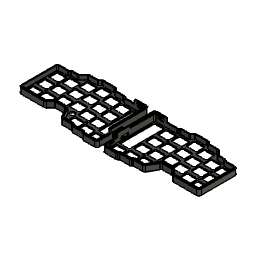
mriya-bumper-fdm-v1.09 (Autodesk Fusion 360 design; units mm, degrees)
Autodesk Fusion 360 part; units mm, degrees
note: some values were not read from the file. Set by a fixed rule: which sketch regions a step uses.
(part 1 of 2)
sketch "mriya" plane through (0, 0, 0) normal (0, 0, 1) x (1, 0, 0)
  line L0 (-101.0213, 15.6719) -> (-94.7787, 21.9145) construction
  line L1 (-26.4858, 1.079) -> (-27.6142, 2.2074) construction
  line L2 (-138.1, 14.7932) -> (-103.1426, 14.7932) construction
  line L3 (-44.0716, 2.7932) -> (-29.0284, 2.7932) construction
  line L4 (-8.6, 0.4932) -> (-25.0716, 0.4932) construction
  line L5 (-64.4741, 6.1094) -> (-72.7517, 20.7608) construction
  line L6 (-45.4858, 3.379) -> (-46.6142, 4.5074) construction
  line L7 (-122.6142, 71.579) -> (-121.4858, 72.7074) construction
  line L8 (-101.0716, 81.2932) -> (-87.2284, 81.2932) construction
  line L9 (-138.1, 70.9932) -> (-124.0284, 70.9932) construction
  line L10 (-92.6574, 22.7932) -> (-76.2344, 22.7932) construction
  line L11 (-48.0284, 5.0932) -> (-62.7328, 5.0932) construction
  line L12 (-82.0716, 84.7932) -> (-64.7284, 84.7932) construction
  line L13 (-58.5716, 80.2932) -> (-45.7284, 80.2932) construction
  line L14 (-24.1, 19.4932) -> (-7.1, 19.4932) construction
  line L15 (-25.6, 20.9932) -> (-25.6, 77.9932) construction
  line L16 (-83.4858, 84.2074) -> (-85.8142, 81.879) construction
  line L17 (-63.3142, 84.2074) -> (-59.9858, 80.879) construction
  line L18 (-139.6, 69.4932) -> (-139.6, 16.2932) construction
  line L19 (-43.1858, 78.579) -> (-44.3142, 79.7074) construction
  line L20 (-99.4, 40.3932) -> (-99.4, 27.9932) construction
  line L21 (-98.6, 41.1932) -> (-86.2, 41.1932) construction
  line L22 (-98.6, 27.1932) -> (-86.2, 27.1932) construction
  line L23 (-85.4, 40.3932) -> (-85.4, 27.9932) construction
  line L24 (-42.4, 56.0932) -> (-42.4, 43.6932) construction
  line L25 (-41.6, 56.8932) -> (-29.2, 56.8932) construction
  line L26 (-41.6, 42.8932) -> (-29.2, 42.8932) construction
  line L27 (-28.4, 56.0932) -> (-28.4, 43.6932) construction
  line L28 (-61.4, 58.3932) -> (-61.4, 45.9932) construction
  line L29 (-60.6, 59.1932) -> (-48.2, 59.1932) construction
  line L30 (-60.6, 45.1932) -> (-48.2, 45.1932) construction
  line L31 (-47.4, 58.3932) -> (-47.4, 45.9932) construction
  line L32 (-137.4, 68.0932) -> (-137.4, 55.6932) construction
  line L33 (-136.6, 68.8932) -> (-124.2, 68.8932) construction
  line L34 (-136.6, 54.8932) -> (-124.2, 54.8932) construction
  line L35 (-123.4, 68.0932) -> (-123.4, 55.6932) construction
  line L36 (-61.4, 39.3932) -> (-61.4, 26.9932) construction
  line L37 (-60.6, 40.1932) -> (-48.2, 40.1932) construction
  line L38 (-60.6, 26.1932) -> (-48.2, 26.1932) construction
  line L39 (-47.4, 39.3932) -> (-47.4, 26.9932) construction
  line L40 (-42.4, 18.0932) -> (-42.4, 5.6932) construction
  line L41 (-41.6, 18.8932) -> (-29.2, 18.8932) construction
  line L42 (-41.6, 4.8932) -> (-29.2, 4.8932) construction
  line L43 (-28.4, 18.0932) -> (-28.4, 5.6932) construction
  line L44 (-23.4, 15.7932) -> (-23.4, 3.3932) construction
  line L45 (-22.6, 16.5932) -> (-10.2, 16.5932) construction
  line L46 (-22.6, 2.5932) -> (-10.2, 2.5932) construction
  line L47 (-9.4, 15.7932) -> (-9.4, 3.3932) construction
  line L48 (-137.4, 49.0932) -> (-137.4, 36.6932) construction
  line L49 (-136.6, 49.8932) -> (-124.2, 49.8932) construction
  line L50 (-136.6, 35.8932) -> (-124.2, 35.8932) construction
  line L51 (-123.4, 49.0932) -> (-123.4, 36.6932) construction
  line L52 (-118.4, 51.3932) -> (-118.4, 38.9932) construction
  line L53 (-117.6, 52.1932) -> (-105.2, 52.1932) construction
  line L54 (-117.6, 38.1932) -> (-105.2, 38.1932) construction
  line L55 (-104.4, 51.3932) -> (-104.4, 38.9932) construction
  line L56 (-137.4, 30.0932) -> (-137.4, 17.6932) construction
  line L57 (-136.6, 30.8932) -> (-124.2, 30.8932) construction
  line L58 (-136.6, 16.8932) -> (-124.2, 16.8932) construction
  line L59 (-123.4, 30.0932) -> (-123.4, 17.6932) construction
  line L60 (-61.4, 20.3932) -> (-61.4, 7.9932) construction
  line L61 (-60.6, 21.1932) -> (-48.2, 21.1932) construction
  line L62 (-60.6, 7.1932) -> (-48.2, 7.1932) construction
  line L63 (-47.4, 20.3932) -> (-47.4, 7.9932) construction
  line L64 (-80.4, 43.8932) -> (-80.4, 31.4932) construction
  line L65 (-79.6, 44.6932) -> (-67.2, 44.6932) construction
  line L66 (-79.6, 30.6932) -> (-67.2, 30.6932) construction
  line L67 (-66.4, 43.8932) -> (-66.4, 31.4932) construction
  line L68 (-80.4, 81.8932) -> (-80.4, 69.4932) construction
  line L69 (-79.6, 82.6932) -> (-67.2, 82.6932) construction
  line L70 (-79.6, 68.6932) -> (-67.2, 68.6932) construction
  line L71 (-66.4, 81.8932) -> (-66.4, 69.4932) construction
  line L72 (-42.4, 37.0932) -> (-42.4, 24.6932) construction
  line L73 (-41.6, 37.8932) -> (-29.2, 37.8932) construction
  line L74 (-41.6, 23.8932) -> (-29.2, 23.8932) construction
  line L75 (-28.4, 37.0932) -> (-28.4, 24.6932) construction
  line L76 (-118.4, 32.3932) -> (-118.4, 19.9932) construction
  line L77 (-117.6, 33.1932) -> (-105.2, 33.1932) construction
  line L78 (-117.6, 19.1932) -> (-105.2, 19.1932) construction
  line L79 (-104.4, 32.3932) -> (-104.4, 19.9932) construction
  line L80 (-61.4, 77.3932) -> (-61.4, 64.9932) construction
  line L81 (-60.6, 78.1932) -> (-48.2, 78.1932) construction
  line L82 (-60.6, 64.1932) -> (-48.2, 64.1932) construction
  line L83 (-47.4, 77.3932) -> (-47.4, 64.9932) construction
  line L84 (-42.4, 75.0932) -> (-42.4, 62.6932) construction
  line L85 (-41.6, 75.8932) -> (-29.2, 75.8932) construction
  line L86 (-41.6, 61.8932) -> (-29.2, 61.8932) construction
  line L87 (-28.4, 75.0932) -> (-28.4, 62.6932) construction
  line L88 (-118.4, 70.3932) -> (-118.4, 57.9932) construction
  line L89 (-117.6, 71.1932) -> (-105.2, 71.1932) construction
  line L90 (-117.6, 57.1932) -> (-105.2, 57.1932) construction
  line L91 (-104.4, 70.3932) -> (-104.4, 57.9932) construction
  line L92 (-99.4, 59.3932) -> (-99.4, 46.9932) construction
  line L93 (-98.6, 60.1932) -> (-86.2, 60.1932) construction
  line L94 (-98.6, 46.1932) -> (-86.2, 46.1932) construction
  line L95 (-85.4, 59.3932) -> (-85.4, 46.9932) construction
  line L96 (-80.4, 62.8932) -> (-80.4, 50.4932) construction
  line L97 (-79.6, 63.6932) -> (-67.2, 63.6932) construction
  line L98 (-79.6, 49.6932) -> (-67.2, 49.6932) construction
  line L99 (-66.4, 62.8932) -> (-66.4, 50.4932) construction
  line L100 (-99.4, 78.3932) -> (-99.4, 65.9932) construction
  line L101 (-98.6, 79.1932) -> (-86.2, 79.1932) construction
  line L102 (-98.6, 65.1932) -> (-86.2, 65.1932) construction
  line L103 (-85.4, 78.3932) -> (-85.4, 65.9932) construction
  circle A0 centre (-120.9, 53.5432) radius 1.75
  circle A1 centre (-120.9, 34.5432) radius 1.75
  circle A2 centre (-68.5, 23.5932) radius 4
  circle A3 centre (-44.9, 22.5432) radius 1.75
  circle A4 centre (-44.9, 60.5432) radius 1.75
  arc A5 (-43.1858, 78.579) -> (-41.7716, 77.9932) centre (-41.7716, 79.9932) ccw construction
  arc A6 (-44.3142, 79.7074) -> (-45.7284, 80.2932) centre (-45.7285, 78.2931) ccw construction
  arc A7 (-59.9858, 80.879) -> (-58.5716, 80.2932) centre (-58.5716, 82.2931) ccw construction
  arc A8 (-63.3142, 84.2074) -> (-64.7284, 84.7932) centre (-64.7285, 82.7931) ccw construction
  arc A9 (-82.0716, 84.7932) -> (-83.4858, 84.2074) centre (-82.0716, 82.7933) ccw construction
  arc A10 (-87.2284, 81.2932) -> (-85.8142, 81.879) centre (-87.2284, 83.2932) ccw construction
  arc A11 (-101.0716, 81.2932) -> (-102.4858, 80.7074) centre (-101.0716, 79.2933) ccw construction
  arc A12 (-120.0716, 73.2932) -> (-121.4858, 72.7074) centre (-120.0716, 71.2933) ccw construction
  arc A13 (-124.0284, 70.9932) -> (-122.6142, 71.579) centre (-124.0284, 72.9932) ccw construction
  arc A14 (-138.1, 70.9932) -> (-139.6, 69.4932) centre (-138.1, 69.4932) ccw construction
  arc A15 (-139.6, 16.2932) -> (-138.1, 14.7932) centre (-138.1, 16.2932) ccw construction
  arc A16 (-103.1426, 14.7932) -> (-101.0213, 15.6719) centre (-103.1426, 17.7931) ccw construction
  arc A17 (-92.6574, 22.7932) -> (-94.7787, 21.9145) centre (-92.6573, 19.7931) ccw construction
  arc A18 (-72.7517, 20.7608) -> (-76.2344, 22.7932) centre (-76.2344, 18.793) ccw construction
  arc A19 (-64.4741, 6.1094) -> (-62.7328, 5.0932) centre (-62.7328, 7.0932) ccw construction
  arc A20 (-46.6142, 4.5074) -> (-48.0284, 5.0932) centre (-48.0284, 3.0933) ccw construction
  arc A21 (-45.4858, 3.379) -> (-44.0716, 2.7932) centre (-44.0715, 4.7933) ccw construction
  arc A22 (-27.6142, 2.2074) -> (-29.0284, 2.7932) centre (-29.0284, 0.7933) ccw construction
  arc A23 (-26.4858, 1.079) -> (-25.0716, 0.4932) centre (-25.0715, 2.4933) ccw construction
  arc A24 (-8.6, 0.4932) -> (-7.1, 1.9932) centre (-8.6, 1.9932) ccw construction
  arc A25 (-25.6, 20.9932) -> (-24.1, 19.4932) centre (-24.1, 20.9932) ccw construction
  line L104 (-7.1, 1.9932) -> (-7.1, 76.4932) construction
  line L105 (-41.7716, 77.9932) -> (-8.6, 77.9932) construction
  arc A26 (-7.1, 76.4932) -> (-8.6, 77.9932) centre (-8.6, 76.4932) ccw construction
  arc A27 (-136.6, 68.8932) -> (-137.4, 68.0932) centre (-136.6, 68.0932) ccw construction
  arc A28 (-123.4, 68.0932) -> (-124.2, 68.8932) centre (-124.2, 68.0932) ccw construction
  arc A29 (-124.2, 54.8932) -> (-123.4, 55.6932) centre (-124.2, 55.6932) ccw construction
  arc A30 (-137.4, 55.6932) -> (-136.6, 54.8932) centre (-136.6, 55.6932) ccw construction
  arc A31 (-136.6, 49.8932) -> (-137.4, 49.0932) centre (-136.6, 49.0932) ccw construction
  arc A32 (-123.4, 49.0932) -> (-124.2, 49.8932) centre (-124.2, 49.0932) ccw construction
  arc A33 (-124.2, 35.8932) -> (-123.4, 36.6932) centre (-124.2, 36.6932) ccw construction
  arc A34 (-137.4, 36.6932) -> (-136.6, 35.8932) centre (-136.6, 36.6932) ccw construction
  arc A35 (-136.6, 30.8932) -> (-137.4, 30.0932) centre (-136.6, 30.0932) ccw construction
  arc A36 (-123.4, 30.0932) -> (-124.2, 30.8932) centre (-124.2, 30.0932) ccw construction
  arc A37 (-124.2, 16.8932) -> (-123.4, 17.6932) centre (-124.2, 17.6932) ccw construction
  arc A38 (-137.4, 17.6932) -> (-136.6, 16.8932) centre (-136.6, 17.6932) ccw construction
  arc A39 (-118.4, 19.9932) -> (-117.6, 19.1932) centre (-117.6, 19.9932) ccw construction
  arc A40 (-105.2, 19.1932) -> (-104.4, 19.9932) centre (-105.2, 19.9932) ccw construction
  arc A41 (-104.4, 32.3932) -> (-105.2, 33.1932) centre (-105.2, 32.3932) ccw construction
  arc A42 (-117.6, 33.1932) -> (-118.4, 32.3932) centre (-117.6, 32.3932) ccw construction
  arc A43 (-105.2, 38.1932) -> (-104.4, 38.9932) centre (-105.2, 38.9932) ccw construction
  arc A44 (-118.4, 38.9932) -> (-117.6, 38.1932) centre (-117.6, 38.9932) ccw construction
  arc A45 (-117.6, 52.1932) -> (-118.4, 51.3932) centre (-117.6, 51.3932) ccw construction
  arc A46 (-104.4, 51.3932) -> (-105.2, 52.1932) centre (-105.2, 51.3932) ccw construction
  arc A47 (-118.4, 57.9932) -> (-117.6, 57.1932) centre (-117.6, 57.9932) ccw construction
  arc A48 (-105.2, 57.1932) -> (-104.4, 57.9932) centre (-105.2, 57.9932) ccw construction
  arc A49 (-104.4, 70.3932) -> (-105.2, 71.1932) centre (-105.2, 70.3932) ccw construction
  arc A50 (-117.6, 71.1932) -> (-118.4, 70.3932) centre (-117.6, 70.3932) ccw construction
  arc A51 (-98.6, 79.1932) -> (-99.4, 78.3932) centre (-98.6, 78.3932) ccw construction
  arc A52 (-85.4, 78.3932) -> (-86.2, 79.1932) centre (-86.2, 78.3932) ccw construction
  arc A53 (-86.2, 65.1932) -> (-85.4, 65.9932) centre (-86.2, 65.9932) ccw construction
  arc A54 (-99.4, 65.9932) -> (-98.6, 65.1932) centre (-98.6, 65.9932) ccw construction
  arc A55 (-98.6, 60.1932) -> (-99.4, 59.3932) centre (-98.6, 59.3932) ccw construction
  arc A56 (-85.4, 59.3932) -> (-86.2, 60.1932) centre (-86.2, 59.3932) ccw construction
  arc A57 (-86.2, 46.1932) -> (-85.4, 46.9932) centre (-86.2, 46.9932) ccw construction
  arc A58 (-99.4, 46.9932) -> (-98.6, 46.1932) centre (-98.6, 46.9932) ccw construction
  arc A59 (-98.6, 41.1932) -> (-99.4, 40.3932) centre (-98.6, 40.3932) ccw construction
  arc A60 (-99.4, 27.9932) -> (-98.6, 27.1932) centre (-98.6, 27.9932) ccw construction
  arc A61 (-86.2, 27.1932) -> (-85.4, 27.9932) centre (-86.2, 27.9932) ccw construction
  arc A62 (-85.4, 40.3932) -> (-86.2, 41.1932) centre (-86.2, 40.3932) ccw construction
  arc A63 (-80.4, 31.4932) -> (-79.6, 30.6932) centre (-79.6, 31.4932) ccw construction
  arc A64 (-79.6, 44.6932) -> (-80.4, 43.8932) centre (-79.6, 43.8932) ccw construction
  arc A65 (-66.4, 43.8932) -> (-67.2, 44.6932) centre (-67.2, 43.8932) ccw construction
  arc A66 (-67.2, 30.6932) -> (-66.4, 31.4932) centre (-67.2, 31.4932) ccw construction
  arc A67 (-67.2, 49.6932) -> (-66.4, 50.4932) centre (-67.2, 50.4932) ccw construction
  arc A68 (-80.4, 50.4932) -> (-79.6, 49.6932) centre (-79.6, 50.4932) ccw construction
  arc A69 (-79.6, 63.6932) -> (-80.4, 62.8932) centre (-79.6, 62.8932) ccw construction
  arc A70 (-66.4, 62.8932) -> (-67.2, 63.6932) centre (-67.2, 62.8932) ccw construction
  arc A71 (-67.2, 68.6932) -> (-66.4, 69.4932) centre (-67.2, 69.4932) ccw construction
  arc A72 (-80.4, 69.4932) -> (-79.6, 68.6932) centre (-79.6, 69.4932) ccw construction
  arc A73 (-79.6, 82.6932) -> (-80.4, 81.8932) centre (-79.6, 81.8932) ccw construction
  arc A74 (-66.4, 81.8932) -> (-67.2, 82.6932) centre (-67.2, 81.8932) ccw construction
  arc A75 (-60.6, 78.1932) -> (-61.4, 77.3932) centre (-60.6, 77.3932) ccw construction
  arc A76 (-61.4, 64.9932) -> (-60.6, 64.1932) centre (-60.6, 64.9932) ccw construction
  arc A77 (-48.2, 64.1932) -> (-47.4, 64.9932) centre (-48.2, 64.9932) ccw construction
  arc A78 (-47.4, 77.3932) -> (-48.2, 78.1932) centre (-48.2, 77.3932) ccw construction
  arc A79 (-47.4, 58.3932) -> (-48.2, 59.1932) centre (-48.2, 58.3932) ccw construction
  arc A80 (-60.6, 59.1932) -> (-61.4, 58.3932) centre (-60.6, 58.3932) ccw construction
  arc A81 (-61.4, 45.9932) -> (-60.6, 45.1932) centre (-60.6, 45.9932) ccw construction
  arc A82 (-48.2, 45.1932) -> (-47.4, 45.9932) centre (-48.2, 45.9932) ccw construction
  arc A83 (-47.4, 39.3932) -> (-48.2, 40.1932) centre (-48.2, 39.3932) ccw construction
  arc A84 (-60.6, 40.1932) -> (-61.4, 39.3932) centre (-60.6, 39.3932) ccw construction
  arc A85 (-61.4, 26.9932) -> (-60.6, 26.1932) centre (-60.6, 26.9932) ccw construction
  arc A86 (-48.2, 26.1932) -> (-47.4, 26.9932) centre (-48.2, 26.9932) ccw construction
  arc A87 (-47.4, 20.3932) -> (-48.2, 21.1932) centre (-48.2, 20.3932) ccw construction
  arc A88 (-60.6, 21.1932) -> (-61.4, 20.3932) centre (-60.6, 20.3932) ccw construction
  arc A89 (-61.4, 7.9932) -> (-60.6, 7.1932) centre (-60.6, 7.9932) ccw construction
  arc A90 (-48.2, 7.1932) -> (-47.4, 7.9932) centre (-48.2, 7.9932) ccw construction
  arc A91 (-42.4, 5.6932) -> (-41.6, 4.8932) centre (-41.6, 5.6932) ccw construction
  arc A92 (-29.2, 4.8932) -> (-28.4, 5.6932) centre (-29.2, 5.6932) ccw construction
  arc A93 (-28.4, 18.0932) -> (-29.2, 18.8932) centre (-29.2, 18.0932) ccw construction
  arc A94 (-41.6, 18.8932) -> (-42.4, 18.0932) centre (-41.6, 18.0932) ccw construction
  arc A95 (-23.4, 3.3932) -> (-22.6, 2.5932) centre (-22.6, 3.3932) ccw construction
  arc A96 (-10.2, 2.5932) -> (-9.4, 3.3932) centre (-10.2, 3.3932) ccw construction
  arc A97 (-9.4, 15.7932) -> (-10.2, 16.5932) centre (-10.2, 15.7932) ccw construction
  arc A98 (-22.6, 16.5932) -> (-23.4, 15.7932) centre (-22.6, 15.7932) ccw construction
  arc A99 (-29.2, 23.8932) -> (-28.4, 24.6932) centre (-29.2, 24.6932) ccw construction
  arc A100 (-42.4, 24.6932) -> (-41.6, 23.8932) centre (-41.6, 24.6932) ccw construction
  arc A101 (-41.6, 37.8932) -> (-42.4, 37.0932) centre (-41.6, 37.0932) ccw construction
  arc A102 (-28.4, 37.0932) -> (-29.2, 37.8932) centre (-29.2, 37.0932) ccw construction
  arc A103 (-29.2, 42.8932) -> (-28.4, 43.6932) centre (-29.2, 43.6932) ccw construction
  arc A104 (-42.4, 43.6932) -> (-41.6, 42.8932) centre (-41.6, 43.6932) ccw construction
  arc A105 (-41.6, 56.8932) -> (-42.4, 56.0932) centre (-41.6, 56.0932) ccw construction
  arc A106 (-28.4, 56.0932) -> (-29.2, 56.8932) centre (-29.2, 56.0932) ccw construction
  arc A107 (-29.2, 61.8932) -> (-28.4, 62.6932) centre (-29.2, 62.6932) ccw construction
  arc A108 (-42.4, 62.6932) -> (-41.6, 61.8932) centre (-41.6, 62.6932) ccw construction
  arc A109 (-41.6, 75.8932) -> (-42.4, 75.0932) centre (-41.6, 75.0932) ccw construction
  arc A110 (-28.4, 75.0932) -> (-29.2, 75.8932) centre (-29.2, 75.0932) ccw construction
  circle A111 centre (-22.6, 22.4932) radius 1.1 construction
  circle A112 centre (-10.1, 22.4932) radius 1.1 construction
  line L106 (-7.7, 39.7932) -> (-7.7, 76.4932)
  line L107 (-102.4858, 80.7074) -> (-109.0213, 74.1719) construction
  line L108 (-120.0716, 73.2932) -> (-111.1426, 73.2932) construction
  arc A113 (-111.1426, 73.2932) -> (-109.0213, 74.1719) centre (-111.1426, 76.2932) ccw construction
  arc A114 (-64.7284, 82.7932) -> (-64.7285, 82.7932) centre (-64.7285, 82.7931) ccw
  arc A115 (-45.7284, 78.2932) -> (-45.7285, 78.2932) centre (-45.7285, 78.2931) ccw
  arc A116 (-25.0716, 2.4932) -> (-25.0715, 2.4932) centre (-25.0715, 2.4933) ccw
  arc A117 (-44.0716, 4.7932) -> (-44.0715, 4.7932) centre (-44.0715, 4.7933) ccw
  line L109 (-138.9, 56.8932) -> (-138.9, 66.8932)
  line L110 (-136.9, 68.8932) -> (-123.9, 68.8932)
  arc A118 (-121.9, 66.8932) -> (-123.9, 68.8932) centre (-123.9, 66.8932) ccw
  arc A119 (-138.9, 56.8932) -> (-136.9, 54.8932) centre (-136.9, 56.8932) ccw
  arc A120 (-136.9, 68.8932) -> (-138.9, 66.8932) centre (-136.9, 66.8932) ccw
  arc A121 (-138.9, 37.8932) -> (-136.9, 35.8932) centre (-136.9, 37.8932) ccw
  line L111 (-138.9, 37.8932) -> (-138.9, 47.8932)
  arc A122 (-136.9, 49.8932) -> (-138.9, 47.8932) centre (-136.9, 47.8932) ccw
  line L112 (-136.9, 49.8932) -> (-123.9, 49.8932)
  arc A123 (-121.9, 47.8932) -> (-123.9, 49.8932) centre (-123.9, 47.8932) ccw
  arc A124 (-123.9, 16.8932) -> (-121.9, 18.8932) centre (-123.9, 18.8932) ccw
  line L113 (-123.9, 16.8932) -> (-136.9, 16.8932)
  arc A125 (-138.9, 18.8932) -> (-136.9, 16.8932) centre (-136.9, 18.8932) ccw
  line L114 (-138.9, 18.8932) -> (-138.9, 28.8932)
  arc A126 (-136.9, 30.8932) -> (-138.9, 28.8932) centre (-136.9, 28.8932) ccw
  line L115 (-136.9, 30.8932) -> (-123.9, 30.8932)
  arc A127 (-121.9, 28.8932) -> (-123.9, 30.8932) centre (-123.9, 28.8932) ccw
  line L116 (-121.9, 28.8932) -> (-121.9, 18.8932)
  arc A128 (-104.9, 57.1932) -> (-102.9, 59.1932) centre (-104.9, 59.1932) ccw
  line L117 (-104.9, 57.1932) -> (-117.9, 57.1932)
  arc A129 (-119.9, 59.1932) -> (-117.9, 57.1932) centre (-117.9, 59.1932) ccw
  line L118 (-119.9, 59.1932) -> (-119.9, 69.1932)
  arc A130 (-117.9, 71.1932) -> (-119.9, 69.1932) centre (-117.9, 69.1932) ccw
  line L119 (-117.9, 71.1932) -> (-104.9, 71.1932)
  arc A131 (-102.9, 69.1932) -> (-104.9, 71.1932) centre (-104.9, 69.1932) ccw
  line L120 (-102.9, 69.1932) -> (-102.9, 59.1932)
  arc A132 (-104.9, 38.1932) -> (-102.9, 40.1932) centre (-104.9, 40.1932) ccw
  line L121 (-104.9, 38.1932) -> (-117.9, 38.1932)
  arc A133 (-119.9, 40.1932) -> (-117.9, 38.1932) centre (-117.9, 40.1932) ccw
  arc A134 (-102.9, 50.1932) -> (-104.9, 52.1932) centre (-104.9, 50.1932) ccw
  line L122 (-102.9, 50.1932) -> (-102.9, 40.1932)
  arc A135 (-104.9, 19.1932) -> (-102.9, 21.1932) centre (-104.9, 21.1932) ccw
  line L123 (-104.9, 19.1932) -> (-117.9, 19.1932)
  arc A136 (-119.9, 21.1932) -> (-117.9, 19.1932) centre (-117.9, 21.1932) ccw
  arc A137 (-102.9, 31.1932) -> (-104.9, 33.1932) centre (-104.9, 31.1932) ccw
  line L124 (-102.9, 31.1932) -> (-102.9, 21.1932)
  arc A138 (-85.9, 65.1932) -> (-83.9, 67.1932) centre (-85.9, 67.1932) ccw
  line L125 (-85.9, 65.1932) -> (-98.9, 65.1932)
  arc A139 (-100.9, 67.1932) -> (-98.9, 65.1932) centre (-98.9, 67.1932) ccw
  line L126 (-100.9, 67.1932) -> (-100.9, 77.1932)
  arc A140 (-98.9, 79.1932) -> (-100.9, 77.1932) centre (-98.9, 77.1932) ccw
  line L127 (-98.9, 79.1932) -> (-85.9, 79.1932)
  arc A141 (-83.9, 77.1932) -> (-85.9, 79.1932) centre (-85.9, 77.1932) ccw
  line L128 (-83.9, 77.1932) -> (-83.9, 67.1932)
  arc A142 (-85.9, 46.1932) -> (-83.9, 48.1932) centre (-85.9, 48.1932) ccw
  line L129 (-85.9, 46.1932) -> (-98.9, 46.1932)
  arc A143 (-100.9, 48.1932) -> (-98.9, 46.1932) centre (-98.9, 48.1932) ccw
  line L130 (-100.9, 48.1932) -> (-100.9, 58.1932)
  arc A144 (-98.9, 60.1932) -> (-100.9, 58.1932) centre (-98.9, 58.1932) ccw
  line L131 (-98.9, 60.1932) -> (-85.9, 60.1932)
  arc A145 (-83.9, 58.1932) -> (-85.9, 60.1932) centre (-85.9, 58.1932) ccw
  line L132 (-83.9, 58.1932) -> (-83.9, 48.1932)
  arc A146 (-85.9, 27.1932) -> (-83.9, 29.1932) centre (-85.9, 29.1932) ccw
  line L133 (-85.9, 27.1932) -> (-98.9, 27.1932)
  arc A147 (-100.9, 29.1932) -> (-98.9, 27.1932) centre (-98.9, 29.1932) ccw
  line L134 (-100.9, 29.1932) -> (-100.9, 39.1932)
  arc A148 (-98.9, 41.1932) -> (-100.9, 39.1932) centre (-98.9, 39.1932) ccw
  line L135 (-98.9, 41.1932) -> (-85.9, 41.1932)
  arc A149 (-83.9, 39.1932) -> (-85.9, 41.1932) centre (-85.9, 39.1932) ccw
  line L136 (-83.9, 39.1932) -> (-83.9, 29.1932)
  arc A150 (-66.9, 30.6932) -> (-64.9, 32.6932) centre (-66.9, 32.6932) ccw
  line L137 (-66.9, 30.6932) -> (-79.9, 30.6932)
  arc A151 (-81.9, 32.6932) -> (-79.9, 30.6932) centre (-79.9, 32.6932) ccw
  line L138 (-81.9, 32.6932) -> (-81.9, 42.6932)
  arc A152 (-79.9, 44.6932) -> (-81.9, 42.6932) centre (-79.9, 42.6932) ccw
  line L139 (-79.9, 44.6932) -> (-66.9, 44.6932)
  arc A153 (-64.9, 42.6932) -> (-66.9, 44.6932) centre (-66.9, 42.6932) ccw
  line L140 (-64.9, 42.6932) -> (-64.9, 32.6932)
  arc A154 (-66.9, 49.6932) -> (-64.9, 51.6932) centre (-66.9, 51.6932) ccw
  line L141 (-66.9, 49.6932) -> (-79.9, 49.6932)
  arc A155 (-81.9, 51.6932) -> (-79.9, 49.6932) centre (-79.9, 51.6932) ccw
  line L142 (-81.9, 51.6932) -> (-81.9, 61.6932)
  arc A156 (-79.9, 63.6932) -> (-81.9, 61.6932) centre (-79.9, 61.6932) ccw
  line L143 (-79.9, 63.6932) -> (-66.9, 63.6932)
  arc A157 (-64.9, 61.6932) -> (-66.9, 63.6932) centre (-66.9, 61.6932) ccw
  line L144 (-64.9, 61.6932) -> (-64.9, 51.6932)
  arc A158 (-66.9, 68.6932) -> (-64.9, 70.6932) centre (-66.9, 70.6932) ccw
  line L145 (-66.9, 68.6932) -> (-79.9, 68.6932)
  arc A159 (-81.9, 70.6932) -> (-79.9, 68.6932) centre (-79.9, 70.6932) ccw
  line L146 (-81.9, 70.6932) -> (-81.9, 80.6932)
  arc A160 (-79.9, 82.6932) -> (-81.9, 80.6932) centre (-79.9, 80.6932) ccw
  line L147 (-79.9, 82.6932) -> (-66.9, 82.6932)
  arc A161 (-64.9, 80.6932) -> (-66.9, 82.6932) centre (-66.9, 80.6932) ccw
  line L148 (-64.9, 80.6932) -> (-64.9, 70.6932)
  arc A162 (-47.9, 26.1932) -> (-45.9, 28.1932) centre (-47.9, 28.1932) ccw
  line L149 (-47.9, 26.1932) -> (-60.9, 26.1932)
  arc A163 (-62.9, 28.1932) -> (-60.9, 26.1932) centre (-60.9, 28.1932) ccw
  line L150 (-62.9, 28.1932) -> (-62.9, 38.1932)
  arc A164 (-60.9, 40.1932) -> (-62.9, 38.1932) centre (-60.9, 38.1932) ccw
  line L151 (-60.9, 40.1932) -> (-47.9, 40.1932)
  arc A165 (-45.9, 38.1932) -> (-47.9, 40.1932) centre (-47.9, 38.1932) ccw
  line L152 (-45.9, 38.1932) -> (-45.9, 28.1932)
  arc A166 (-47.9, 45.1932) -> (-45.9, 47.1932) centre (-47.9, 47.1932) ccw
  line L153 (-47.9, 45.1932) -> (-60.9, 45.1932)
  arc A167 (-62.9, 47.1932) -> (-60.9, 45.1932) centre (-60.9, 47.1932) ccw
  line L154 (-62.9, 47.1932) -> (-62.9, 57.1932)
  arc A168 (-60.9, 59.1932) -> (-62.9, 57.1932) centre (-60.9, 57.1932) ccw
  arc A169 (-47.9, 64.1932) -> (-45.9, 66.1932) centre (-47.9, 66.1932) ccw
  line L155 (-47.9, 64.1932) -> (-60.9, 64.1932)
  arc A170 (-62.9, 66.1932) -> (-60.9, 64.1932) centre (-60.9, 66.1932) ccw
  line L156 (-62.9, 66.1932) -> (-62.9, 76.1932)
  arc A171 (-60.9, 78.1932) -> (-62.9, 76.1932) centre (-60.9, 76.1932) ccw
  line L157 (-60.9, 78.1932) -> (-47.9, 78.1932)
  arc A172 (-45.9, 76.1932) -> (-47.9, 78.1932) centre (-47.9, 76.1932) ccw
  line L158 (-45.9, 76.1932) -> (-45.9, 66.1932)
  arc A173 (-47.9, 7.1932) -> (-45.9, 9.1932) centre (-47.9, 9.1932) ccw
  line L159 (-47.9, 7.1932) -> (-60.9, 7.1932)
  arc A174 (-62.9, 9.1932) -> (-60.9, 7.1932) centre (-60.9, 9.1932) ccw
  line L160 (-62.9, 9.1932) -> (-62.9, 19.1932)
  arc A175 (-60.9, 21.1932) -> (-62.9, 19.1932) centre (-60.9, 19.1932) ccw
  arc A176 (-28.9, 4.8932) -> (-26.9, 6.8932) centre (-28.9, 6.8932) ccw
  line L161 (-28.9, 4.8932) -> (-41.9, 4.8932)
  arc A177 (-43.9, 6.8932) -> (-41.9, 4.8932) centre (-41.9, 6.8932) ccw
  line L162 (-43.9, 6.8932) -> (-43.9, 16.8932)
  arc A178 (-41.9, 18.8932) -> (-43.9, 16.8932) centre (-41.9, 16.8932) ccw
  line L163 (-41.9, 18.8932) -> (-28.9, 18.8932)
  arc A179 (-26.9, 16.8932) -> (-28.9, 18.8932) centre (-28.9, 16.8932) ccw
  line L164 (-26.9, 16.8932) -> (-26.9, 6.8932)
  arc A180 (-28.9, 23.8932) -> (-26.9, 25.8932) centre (-28.9, 25.8932) ccw
  arc A181 (-41.9, 37.8932) -> (-43.9, 35.8932) centre (-41.9, 35.8932) ccw
  line L165 (-41.9, 37.8932) -> (-28.9, 37.8932)
  arc A182 (-26.9, 35.8932) -> (-28.9, 37.8932) centre (-28.9, 35.8932) ccw
  line L166 (-26.9, 35.8932) -> (-26.9, 25.8932)
  arc A183 (-28.9, 42.8932) -> (-26.9, 44.8932) centre (-28.9, 44.8932) ccw
  line L167 (-28.9, 42.8932) -> (-41.9, 42.8932)
  arc A184 (-43.9, 44.8932) -> (-41.9, 42.8932) centre (-41.9, 44.8932) ccw
  line L168 (-43.9, 44.8932) -> (-43.9, 54.8932)
  arc A185 (-41.9, 56.8932) -> (-43.9, 54.8932) centre (-41.9, 54.8932) ccw
  line L169 (-41.9, 56.8932) -> (-28.9, 56.8932)
  arc A186 (-26.9, 54.8932) -> (-28.9, 56.8932) centre (-28.9, 54.8932) ccw
  line L170 (-26.9, 54.8932) -> (-26.9, 44.8932)
  arc A187 (-28.9, 61.8932) -> (-26.9, 63.8932) centre (-28.9, 63.8932) ccw
  arc A188 (-41.9, 75.8932) -> (-43.9, 73.8932) centre (-41.9, 73.8932) ccw
  line L171 (-41.9, 75.8932) -> (-28.9, 75.8932)
  arc A189 (-26.9, 73.8932) -> (-28.9, 75.8932) centre (-28.9, 73.8932) ccw
  line L172 (-26.9, 73.8932) -> (-26.9, 63.8932)
  arc A190 (-9.9, 2.5932) -> (-7.9, 4.5932) centre (-9.9, 4.5932) ccw
  line L173 (-9.9, 2.5932) -> (-22.9, 2.5932)
  arc A191 (-24.9, 4.5932) -> (-22.9, 2.5932) centre (-22.9, 4.5932) ccw
  line L174 (-24.9, 4.5932) -> (-24.9, 14.5932)
  arc A192 (-22.9, 16.5932) -> (-24.9, 14.5932) centre (-22.9, 14.5932) ccw
  line L175 (-22.9, 16.5932) -> (-9.9, 16.5932)
  arc A193 (-7.9, 14.5932) -> (-9.9, 16.5932) centre (-9.9, 14.5932) ccw
  line L176 (-7.9, 14.5932) -> (-7.9, 4.5932)
  arc A194 (-9.9, 19.8932) -> (-7.9, 21.8932) centre (-9.9, 21.8932) ccw
  line L177 (-9.9, 19.8932) -> (-22.9, 19.8932)
  arc A195 (-24.9, 21.8932) -> (-22.9, 19.8932) centre (-22.9, 21.8932) ccw
  line L178 (-24.9, 21.8932) -> (-24.9, 73.8932)
  arc A196 (-22.9, 75.8932) -> (-24.9, 73.8932) centre (-22.9, 73.8932) ccw
  line L179 (-22.9, 75.8932) -> (-9.9, 75.8932)
  arc A197 (-7.9, 73.8932) -> (-9.9, 75.8932) centre (-9.9, 73.8932) ccw
  line L180 (-7.9, 73.8932) -> (-7.9, 21.8932)
  line L181 (-25.8, 78.1932) -> (-25.8, 80.6932)
  line L182 (-6.9, 19.2932) -> (-4.4, 19.2932)
  line L183 (-121.9, 47.8932) -> (-121.9, 38.3145)
  line L184 (-124.3213, 35.8932) -> (-136.9, 35.8932)
  line L185 (-117.4787, 33.1932) -> (-104.9, 33.1932)
  line L186 (-119.9, 21.1932) -> (-119.9, 30.7719)
  line L187 (-123.2607, 36.3325) -> (-122.3393, 37.2539)
  line L188 (-118.5393, 32.7539) -> (-119.4607, 31.8325)
  line L189 (-121.9, 66.8932) -> (-121.9, 57.3145)
  line L190 (-124.3213, 54.8932) -> (-136.9, 54.8932)
  line L191 (-117.4787, 52.1932) -> (-104.9, 52.1932)
  line L192 (-119.9, 40.1932) -> (-119.9, 49.7719)
  line L193 (-123.2607, 55.3325) -> (-122.3393, 56.2539)
  line L194 (-118.5393, 51.7539) -> (-119.4607, 50.8325)
  arc A198 (-122.3393, 56.2539) -> (-121.9, 57.3145) centre (-123.4, 57.3145) ccw
  arc A199 (-124.3213, 54.8932) -> (-123.2607, 55.3325) centre (-124.3213, 56.3932) ccw
  arc A200 (-117.4787, 52.1932) -> (-118.5393, 51.7539) centre (-117.4787, 50.6932) ccw
  arc A201 (-119.4607, 50.8325) -> (-119.9, 49.7719) centre (-118.4, 49.7719) ccw
  arc A202 (-124.3213, 35.8932) -> (-123.2607, 36.3325) centre (-124.3213, 37.3932) ccw
  arc A203 (-122.3393, 37.2539) -> (-121.9, 38.3145) centre (-123.4, 38.3145) ccw
  arc A204 (-119.4607, 31.8325) -> (-119.9, 30.7719) centre (-118.4, 30.7719) ccw
  arc A205 (-117.4787, 33.1932) -> (-118.5393, 32.7539) centre (-117.4787, 31.6932) ccw
  line L195 (-43.9, 64.3145) -> (-43.9, 73.8932)
  line L196 (-28.9, 61.8932) -> (-41.4787, 61.8932)
  line L197 (-60.9, 59.1932) -> (-48.3213, 59.1932)
  line L198 (-45.9, 56.7719) -> (-45.9, 47.1932)
  line L199 (-47.2607, 58.7539) -> (-46.3393, 57.8325)
  line L200 (-42.5393, 62.3325) -> (-43.4607, 63.2539)
  arc A206 (-47.2607, 58.7539) -> (-48.3213, 59.1932) centre (-48.3213, 57.6932) ccw
  arc A207 (-45.9, 56.7719) -> (-46.3393, 57.8325) centre (-47.4, 56.7719) ccw
  arc A208 (-43.9, 64.3145) -> (-43.4607, 63.2539) centre (-42.4, 64.3145) ccw
  arc A209 (-42.5393, 62.3325) -> (-41.4787, 61.8932) centre (-41.4787, 63.3932) ccw
  line L201 (-43.9, 26.3145) -> (-43.9, 35.8932)
  line L202 (-28.9, 23.8932) -> (-41.4787, 23.8932)
  line L203 (-60.9, 21.1932) -> (-48.3213, 21.1932)
  line L204 (-45.9, 18.7719) -> (-45.9, 9.1932)
  line L205 (-47.2607, 20.7539) -> (-46.3393, 19.8325)
  line L206 (-42.5393, 24.3325) -> (-43.4607, 25.2539)
  arc A210 (-47.2607, 20.7539) -> (-48.3213, 21.1932) centre (-48.3213, 19.6932) ccw
  arc A211 (-45.9, 18.7719) -> (-46.3393, 19.8325) centre (-47.4, 18.7719) ccw
  arc A212 (-43.9, 26.3145) -> (-43.4607, 25.2539) centre (-42.4, 26.3145) ccw
  arc A213 (-42.5393, 24.3325) -> (-41.4787, 23.8932) centre (-41.4787, 25.3932) ccw
  line L207 (-138.1, 14.5932) -> (-103.1426, 14.5932)
  arc A214 (-103.1426, 14.5932) -> (-100.8799, 15.5305) centre (-103.1426, 17.7931) ccw
  line L208 (-100.8799, 15.5305) -> (-94.6373, 21.7731)
  arc A215 (-92.6574, 22.5932) -> (-94.6373, 21.7731) centre (-92.6573, 19.7931) ccw
  line L209 (-92.6574, 22.5932) -> (-76.2344, 22.5932)
  arc A216 (-72.9258, 20.6624) -> (-76.2344, 22.5932) centre (-76.2344, 18.793) ccw
  line L210 (-64.6482, 6.011) -> (-72.9258, 20.6624)
  arc A217 (-64.6482, 6.011) -> (-62.7328, 4.8932) centre (-62.7328, 7.0932) ccw
  line L211 (-48.0284, 4.8932) -> (-62.7328, 4.8932)
  arc A218 (-46.7556, 4.366) -> (-48.0284, 4.8932) centre (-48.0284, 3.0933) ccw
  line L212 (-45.6272, 3.2376) -> (-46.7556, 4.366)
  arc A219 (-45.6272, 3.2376) -> (-44.0716, 2.5932) centre (-44.0715, 4.7933) ccw
  line L213 (-44.0716, 2.5932) -> (-29.0284, 2.5932)
  arc A220 (-27.7556, 2.066) -> (-29.0284, 2.5932) centre (-29.0284, 0.7933) ccw
  line L214 (-26.6272, 0.9376) -> (-27.7556, 2.066)
  arc A221 (-26.6272, 0.9376) -> (-25.0716, 0.2932) centre (-25.0715, 2.4933) ccw
  line L215 (-8.6, 0.2932) -> (-25.0716, 0.2932)
  arc A222 (-8.6, 0.2932) -> (-6.9, 1.9932) centre (-8.6, 1.9932) ccw
  line L216 (-6.9, 1.9932) -> (-6.9, 76.4932)
  arc A223 (-6.9, 76.4932) -> (-8.6, 78.1932) centre (-8.6, 76.4932) ccw
  line L217 (-41.7716, 78.1932) -> (-8.6, 78.1932)
  arc A224 (-43.0444, 78.7204) -> (-41.7716, 78.1932) centre (-41.7716, 79.9932) ccw
  line L218 (-43.0444, 78.7204) -> (-44.1728, 79.8488)
  arc A225 (-44.1728, 79.8488) -> (-45.7284, 80.4932) centre (-45.7285, 78.2931) ccw
  line L219 (-58.5716, 80.4932) -> (-45.7284, 80.4932)
  arc A226 (-59.8444, 81.0204) -> (-58.5716, 80.4932) centre (-58.5716, 82.2931) ccw
  line L220 (-63.1728, 84.3488) -> (-59.8444, 81.0204)
  arc A227 (-63.1728, 84.3488) -> (-64.7284, 84.9932) centre (-64.7285, 82.7931) ccw
  line L221 (-82.0716, 84.9932) -> (-64.7284, 84.9932)
  arc A228 (-82.0716, 84.9932) -> (-83.6272, 84.3488) centre (-82.0716, 82.7933) ccw
  line L222 (-83.6272, 84.3488) -> (-85.9556, 82.0204)
  arc A229 (-87.2284, 81.4932) -> (-85.9556, 82.0204) centre (-87.2284, 83.2932) ccw
  line L223 (-101.0716, 81.4932) -> (-87.2284, 81.4932)
  arc A230 (-101.0716, 81.4932) -> (-102.6272, 80.8488) centre (-101.0716, 79.2933) ccw
  line L224 (-102.6272, 80.8488) -> (-109.1627, 74.3133)
  arc A231 (-111.1426, 73.4932) -> (-109.1627, 74.3133) centre (-111.1426, 76.2932) ccw
  line L225 (-120.0716, 73.4932) -> (-111.1426, 73.4932)
  arc A232 (-120.0716, 73.4932) -> (-121.6272, 72.8488) centre (-120.0716, 71.2933) ccw
  line L226 (-122.7556, 71.7204) -> (-121.6272, 72.8488)
  arc A233 (-124.0284, 71.1932) -> (-122.7556, 71.7204) centre (-124.0284, 72.9932) ccw
  line L227 (-138.1, 71.1932) -> (-124.0284, 71.1932)
  arc A234 (-138.1, 71.1932) -> (-139.8, 69.4932) centre (-138.1, 69.4932) ccw
  line L228 (-139.8, 69.4932) -> (-139.8, 16.2932)
  arc A235 (-139.8, 16.2932) -> (-138.1, 14.5932) centre (-138.1, 16.2932) ccw
  arc A236 (-7.7, 39.7932) -> (-6.9, 38.9932) centre (-6.9, 39.7932) ccw
  arc A237 (-21.1, 78.1932) -> (-20.3, 77.3932) centre (-20.3, 78.1932) ccw
  line L229 (-20.3, 77.3932) -> (-8.6, 77.3932)
  arc A238 (-7.7, 76.4932) -> (-8.6, 77.3932) centre (-8.6, 76.4932) ccw
  line L230 (-82.7757, 87.4932) -> (-64.0243, 87.4932)
  line L231 (-84.8971, 86.6145) -> (-87.2255, 84.2861)
  line L232 (-101.7757, 83.9932) -> (-87.9326, 83.9932)
  line L233 (-103.8971, 83.1145) -> (-110.579, 76.4325)
  line L234 (-120.7757, 75.9932) -> (-111.6397, 75.9932)
  line L235 (-124.0255, 73.9861) -> (-122.8971, 75.1145)
  line L236 (-138.3, 73.6932) -> (-124.7326, 73.6932)
  line L237 (-142.3, 69.6932) -> (-142.3, 16.0932)
  line L238 (-138.3, 12.0932) -> (-102.6456, 12.0932)
  line L239 (-99.4636, 13.4112) -> (-93.3674, 19.5074)
  line L240 (-91.9532, 20.0932) -> (-77.2264, 20.0932)
  line L241 (-66.4804, 4.1716) -> (-74.6144, 18.5689)
  line L242 (-48.7326, 2.3932) -> (-63.4331, 2.3932)
  line L243 (-44.7757, 0.0932) -> (-29.7326, 0.0932)
  line L244 (-8.4, -2.2068) -> (-25.7757, -2.2068)
  line L245 (-4.4, 1.7932) -> (-4.4, 76.6932)
  line L246 (-41.0674, 80.6932) -> (-8.4, 80.6932)
  line L247 (-41.7745, 80.9861) -> (-42.9029, 82.1145)
  line L248 (-57.8674, 82.9932) -> (-45.0243, 82.9932)
  line L249 (-61.9029, 86.6145) -> (-58.5745, 83.2861)
  line L250 (-27.8971, -1.3281) -> (-29.0255, -0.1997)
  line L251 (-46.8971, 0.9719) -> (-48.0255, 2.1003)
  arc A239 (-138.3, 73.6932) -> (-142.3, 69.6932) centre (-138.3, 69.6932) ccw
  arc A240 (-142.3, 16.0932) -> (-138.3, 12.0932) centre (-138.3, 16.0932) ccw
  arc A241 (-4.4, 76.6932) -> (-8.4, 80.6932) centre (-8.4, 76.6932) ccw
  arc A242 (-8.4, -2.2068) -> (-4.4, 1.7932) centre (-8.4, 1.7932) ccw
  arc A243 (-124.7326, 73.6932) -> (-124.0255, 73.9861) centre (-124.7326, 74.6932) ccw
  arc A244 (-120.7757, 75.9932) -> (-122.8971, 75.1145) centre (-120.7757, 72.9932) ccw
  arc A245 (-111.6397, 75.9932) -> (-110.579, 76.4325) centre (-111.6397, 77.4932) ccw
  arc A246 (-101.7757, 83.9932) -> (-103.8971, 83.1145) centre (-101.7757, 80.9932) ccw
  arc A247 (-87.9326, 83.9932) -> (-87.2255, 84.2861) centre (-87.9326, 84.9932) ccw
  arc A248 (-82.7757, 87.4932) -> (-84.8971, 86.6145) centre (-82.7757, 84.4932) ccw
  arc A249 (-61.9029, 86.6145) -> (-64.0243, 87.4932) centre (-64.0243, 84.4932) ccw
  arc A250 (-58.5745, 83.2861) -> (-57.8674, 82.9932) centre (-57.8674, 83.9932) ccw
  arc A251 (-42.9029, 82.1145) -> (-45.0243, 82.9932) centre (-45.0243, 79.9932) ccw
  arc A252 (-41.7745, 80.9861) -> (-41.0674, 80.6932) centre (-41.0674, 81.6932) ccw
  arc A253 (-27.8971, -1.3281) -> (-25.7757, -2.2068) centre (-25.7757, 0.7932) ccw
  arc A254 (-29.0255, -0.1997) -> (-29.7326, 0.0932) centre (-29.7326, -0.9068) ccw
  arc A255 (-46.8971, 0.9719) -> (-44.7757, 0.0932) centre (-44.7757, 3.0932) ccw
  arc A256 (-48.0255, 2.1003) -> (-48.7326, 2.3932) centre (-48.7326, 1.3932) ccw
  arc A257 (-66.4804, 4.1716) -> (-63.4331, 2.3932) centre (-63.4331, 5.8932) ccw
  arc A258 (-74.6144, 18.5689) -> (-77.2264, 20.0932) centre (-77.2264, 17.0932) ccw
  arc A259 (-91.9532, 20.0932) -> (-93.3674, 19.5074) centre (-91.9532, 18.0932) ccw
  arc A260 (-102.6456, 12.0932) -> (-99.4636, 13.4112) centre (-102.6456, 16.5932) ccw
  line L252 (-7.7, 12.7932) -> (-7.7, 6.3932)
  arc A261 (-7.7, 6.3932) -> (-6.9, 5.5932) centre (-6.9, 6.3932) ccw
  arc A262 (-6.9, 13.5932) -> (-7.7, 12.7932) centre (-6.9, 12.7932) ccw
  dimension "d1" = 3.5
  dimension "d2" = 3.5
  dimension "d3" = 8
  dimension "d4" = 3.5
  dimension "d5" = 3.5
  dimension "d9" = 2.2
  dimension "d12" = 2.2
  constraint tangent L19 A5
  constraint tangent L19 A6
  constraint tangent L13 A7
  constraint tangent L17 A8
  constraint tangent L12 A9
  constraint tangent L16 A10
  constraint tangent L8 A11
  constraint tangent L7 A13
  constraint tangent L9 A14
  constraint tangent L18 A15
  constraint tangent L2 A16
  constraint tangent L0 A17
  constraint tangent L10 A18
  constraint tangent L5 A19
  constraint tangent L11 A20
  constraint tangent L6 A21
  constraint tangent L3 A22
  constraint tangent L1 A23
  constraint tangent L4 A24
  constraint tangent L15 A25
  constraint tangent A24 L104
  constraint perpendicular L104 L105
  constraint tangent L104 A26
  constraint tangent L105 A26
  constraint coincident L15.end L105
  constraint perpendicular L15 L105
  constraint coincident L14.end L104
  constraint perpendicular L14 L104
  constraint tangent L32 A27
  constraint tangent L33 A28
  constraint tangent L35 A29
  constraint tangent L34 A30
  constraint tangent L49 A31
  constraint tangent L49 A32
  constraint tangent L51 A33
  constraint tangent L50 A34
  constraint tangent L57 A35
  constraint tangent L57 A36
  constraint tangent L59 A37
  constraint tangent L58 A38
  constraint tangent L76 A39
  constraint tangent L78 A40
  constraint tangent L79 A41
  constraint tangent L77 A42
  constraint tangent L54 A43
  constraint tangent L54 A44
  constraint tangent L52 A45
  constraint tangent L53 A46
  constraint tangent L90 A47
  constraint tangent L90 A48
  constraint tangent L91 A48
  constraint tangent L91 A49
  constraint tangent L89 A50
  constraint tangent L100 A51
  constraint tangent L101 A52
  constraint tangent L103 A53
  constraint tangent L102 A54
  constraint tangent L93 A55
  constraint tangent L93 A56
  constraint tangent L95 A57
  constraint tangent L94 A58
  constraint tangent L21 A59
  constraint tangent L20 A60
  constraint tangent L22 A60
  constraint tangent L22 A61
  constraint tangent L23 A62
  constraint tangent L64 A63
  constraint tangent L66 A63
  constraint tangent L64 A64
  constraint tangent L65 A65
  constraint tangent L67 A66
  constraint tangent L98 A67
  constraint tangent L98 A68
  constraint tangent L96 A69
  constraint tangent L97 A70
  constraint tangent L70 A71
  constraint tangent L70 A72
  constraint tangent L68 A73
  constraint tangent L69 A74
  constraint tangent L80 A75
  constraint tangent L80 A76
  constraint tangent L82 A76
  constraint tangent L82 A77
  constraint tangent L83 A77
  constraint tangent L83 A78
  constraint tangent L81 A78
  constraint tangent L29 A79
  constraint tangent L29 A80
  constraint tangent L28 A81
  constraint tangent L30 A82
  constraint tangent L37 A83
  constraint tangent L37 A84
  constraint tangent L36 A84
  constraint tangent L36 A85
  constraint tangent L38 A85
  constraint tangent L38 A86
  constraint tangent L39 A86
  constraint tangent L61 A87
  constraint tangent L61 A88
  constraint tangent L60 A88
  constraint tangent L60 A89
  constraint tangent L62 A90
  constraint tangent L40 A91
  constraint tangent L42 A92
  constraint tangent L43 A93
  constraint tangent L41 A93
  constraint tangent L41 A94
  constraint tangent L40 A94
  constraint tangent L44 A95
  constraint tangent L46 A95
  constraint tangent L46 A96
  constraint tangent L47 A96
  constraint tangent L47 A97
  constraint tangent L45 A97
  constraint tangent L45 A98
  constraint tangent L44 A98
  constraint tangent L74 A99
  constraint tangent L75 A99
  constraint tangent L74 A100
  constraint tangent L72 A101
  constraint tangent L73 A102
  constraint tangent L26 A103
  constraint tangent L27 A103
  constraint tangent L26 A104
  constraint tangent L24 A105
  constraint tangent L25 A106
  constraint tangent L86 A107
  constraint tangent L87 A107
  constraint tangent L86 A108
  constraint tangent L84 A109
  constraint tangent L85 A110
  constraint tangent A12 L108
  constraint tangent L107 A113
  constraint tangent L108 A113
  constraint concentric A8 A114
  constraint concentric A6 A115
  constraint concentric A23 A116
  constraint concentric A21 A117
  constraint parallel L109 L189
  constraint tangent A118 L189
  constraint tangent L110 A118
  constraint tangent L109 A119
  constraint tangent L109 A120
  constraint tangent L110 A120
  constraint parallel L111 L183
  constraint tangent A123 L183
  constraint tangent L112 A123
  constraint tangent A121 L111
  constraint tangent L111 A122
  constraint tangent A122 L112
  constraint horizontal L113
  constraint perpendicular L113 L114
  constraint parallel L113 L115
  constraint parallel L114 L116
  constraint tangent A127 L116
  constraint tangent L115 A127
  constraint tangent A124 L113
  constraint tangent A124 L116
  constraint tangent L113 A125
  constraint tangent A125 L114
  constraint tangent L114 A126
  constraint tangent A126 L115
  constraint horizontal L117
  constraint perpendicular L117 L118
  constraint parallel L117 L119
  constraint parallel L118 L120
  constraint tangent A131 L120
  constraint tangent L119 A131
  constraint tangent A128 L117
  constraint tangent A128 L120
  constraint tangent L117 A129
  constraint tangent A129 L118
  constraint tangent L118 A130
  constraint tangent A130 L119
  constraint horizontal L121
  constraint perpendicular L121 L192
  constraint parallel L122 L192
  constraint tangent A134 L122
  constraint tangent A132 L121
  constraint tangent A132 L122
  constraint tangent L121 A133
  constraint tangent A133 L192
  constraint horizontal L123
  constraint perpendicular L123 L186
  constraint parallel L124 L186
  constraint tangent A137 L124
  constraint tangent A135 L123
  constraint tangent A135 L124
  constraint tangent L123 A136
  constraint tangent A136 L186
  constraint horizontal L125
  constraint perpendicular L125 L126
  constraint parallel L125 L127
  constraint parallel L126 L128
  constraint tangent A141 L128
  constraint tangent L127 A141
  constraint tangent A138 L125
  constraint tangent A138 L128
  constraint tangent L125 A139
  constraint tangent A139 L126
  constraint tangent L126 A140
  constraint tangent A140 L127
  constraint horizontal L129
  constraint perpendicular L129 L130
  constraint parallel L129 L131
  constraint parallel L130 L132
  constraint tangent A145 L132
  constraint tangent L131 A145
  constraint tangent A142 L129
  constraint tangent A142 L132
  constraint tangent L129 A143
  constraint tangent A143 L130
  constraint tangent L130 A144
  constraint tangent A144 L131
  constraint horizontal L133
  constraint perpendicular L133 L134
  constraint parallel L133 L135
  constraint parallel L134 L136
  constraint tangent A149 L136
  constraint tangent L135 A149
  constraint tangent A146 L133
  constraint tangent A146 L136
  constraint tangent L133 A147
  constraint tangent A147 L134
  constraint tangent L134 A148
  constraint tangent A148 L135
  constraint horizontal L145
  constraint perpendicular L145 L146
  constraint parallel L145 L147
  constraint parallel L146 L148
  constraint tangent A161 L148
  constraint tangent L147 A161
  constraint tangent A158 L145
  constraint tangent A158 L148
  constraint tangent L145 A159
  constraint tangent A159 L146
  constraint tangent L146 A160
  constraint tangent A160 L147
  constraint horizontal L141
  constraint perpendicular L141 L142
  constraint parallel L141 L143
  constraint parallel L142 L144
  constraint tangent A157 L144
  constraint tangent L143 A157
  constraint tangent A154 L141
  constraint tangent A154 L144
  constraint tangent L141 A155
  constraint tangent A155 L142
  constraint tangent L142 A156
  constraint tangent A156 L143
  constraint horizontal L137
  constraint perpendicular L137 L138
  constraint parallel L137 L139
  constraint parallel L138 L140
  constraint tangent A153 L140
  constraint tangent L139 A153
  constraint tangent A150 L137
  constraint tangent A150 L140
  constraint tangent L137 A151
  constraint tangent A151 L138
  constraint tangent L138 A152
  constraint tangent A152 L139
  constraint horizontal L155
  constraint perpendicular L155 L156
  constraint parallel L155 L157
  constraint parallel L156 L158
  constraint tangent A172 L158
  constraint tangent L157 A172
  constraint tangent A169 L155
  constraint tangent A169 L158
  constraint tangent L155 A170
  constraint tangent A170 L156
  constraint tangent L156 A171
  constraint tangent A171 L157
  constraint horizontal L153
  constraint perpendicular L153 L154
  constraint parallel L153 L197
  constraint tangent A166 L153
  constraint tangent L153 A167
  constraint tangent A167 L154
  constraint tangent L154 A168
  constraint tangent A168 L197
  constraint horizontal L149
  constraint perpendicular L149 L150
  constraint parallel L149 L151
  constraint parallel L150 L152
  constraint tangent A165 L152
  constraint tangent L151 A165
  constraint tangent A162 L149
  constraint tangent A162 L152
  constraint tangent L149 A163
  constraint tangent A163 L150
  constraint tangent L150 A164
  constraint tangent A164 L151
  constraint horizontal L159
  constraint perpendicular L159 L160
  constraint parallel L159 L203
  constraint tangent A173 L159
  constraint tangent L159 A174
  constraint tangent A174 L160
  constraint tangent L160 A175
  constraint tangent A175 L203
  constraint horizontal L196
  constraint parallel L171 L196
  constraint tangent A189 L172
  constraint tangent L171 A189
  constraint tangent A187 L196
  constraint tangent A187 L172
  constraint tangent A188 L171
  constraint horizontal L167
  constraint perpendicular L167 L168
  constraint parallel L167 L169
  constraint parallel L168 L170
  constraint tangent A186 L170
  constraint tangent L169 A186
  constraint tangent A183 L167
  constraint tangent A183 L170
  constraint tangent L167 A184
  constraint tangent A184 L168
  constraint tangent L168 A185
  constraint tangent A185 L169
  constraint horizontal L202
  constraint parallel L165 L202
  constraint tangent A182 L166
  constraint tangent L165 A182
  constraint tangent A180 L202
  constraint tangent A180 L166
  constraint tangent A181 L165
  constraint horizontal L161
  constraint perpendicular L161 L162
  constraint parallel L161 L163
  constraint parallel L162 L164
  constraint tangent A179 L164
  constraint tangent L163 A179
  constraint tangent A176 L161
  constraint tangent A176 L164
  constraint tangent L161 A177
  constraint tangent A177 L162
  constraint tangent L162 A178
  constraint tangent A178 L163
  constraint horizontal L173
  constraint perpendicular L173 L174
  constraint parallel L173 L175
  constraint parallel L174 L176
  constraint tangent A193 L176
  constraint tangent L175 A193
  constraint tangent A190 L173
  constraint tangent A190 L176
  constraint tangent L173 A191
  constraint tangent A191 L174
  constraint tangent L174 A192
  constraint tangent A192 L175
  constraint horizontal L177
  constraint perpendicular L177 L178
  constraint parallel L177 L179
  constraint parallel L178 L180
  constraint tangent A197 L180
  constraint tangent L179 A197
  constraint tangent A194 L177
  constraint tangent A194 L180
  constraint tangent L177 A195
  constraint tangent A195 L178
  constraint tangent L178 A196
  constraint tangent A196 L179
  constraint parallel L187 L188
  constraint parallel L193 L194
  constraint tangent L189 A198
  constraint tangent L193 A198
  constraint tangent L190 A199
  constraint tangent L193 A199
  constraint tangent L191 A200
  constraint tangent L194 A200
  constraint tangent L192 A201
  constraint tangent L194 A201
  constraint tangent L184 A202
  constraint tangent L187 A202
  constraint tangent L183 A203
  constraint tangent L187 A203
  constraint tangent L186 A204
  constraint tangent L188 A204
  constraint tangent L185 A205
  constraint tangent L188 A205
  constraint parallel L199 L200
  constraint tangent L197 A206
  constraint tangent L199 A206
  constraint tangent L198 A207
  constraint tangent L199 A207
  constraint tangent L195 A208
  constraint tangent L200 A208
  constraint tangent L196 A209
  constraint tangent L200 A209
  constraint parallel L205 L206
  constraint tangent L203 A210
  constraint tangent L205 A210
  constraint tangent L204 A211
  constraint tangent L205 A211
  constraint tangent L201 A212
  constraint tangent L206 A212
  constraint tangent L202 A213
  constraint tangent L206 A213
  constraint coincident L217 L181.start
  constraint coincident L216 L182.start
  constraint tangent L106 A236
  constraint tangent A237 L229
  constraint tangent L229 A238
  constraint tangent L106 A238
  constraint coincident L246 L181.end
  constraint coincident L245 L182.end
  constraint tangent L236 A239
  constraint tangent L237 A239
  constraint tangent L237 A240
  constraint tangent L238 A240
  constraint tangent L246 A241
  constraint tangent L245 A241
  constraint tangent L245 A242
  constraint tangent L244 A242
  constraint tangent L235 A243
  constraint tangent L236 A243
  constraint tangent L234 A244
  constraint tangent L235 A244
  constraint tangent L233 A245
  constraint tangent L234 A245
  constraint tangent L232 A246
  constraint tangent L233 A246
  constraint tangent L231 A247
  constraint tangent L232 A247
  constraint tangent L230 A248
  constraint tangent L231 A248
  constraint tangent L230 A249
  constraint tangent L249 A249
  constraint tangent L248 A250
  constraint tangent L249 A250
  constraint tangent L248 A251
  constraint tangent L247 A251
  constraint tangent L246 A252